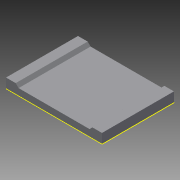
# Autodesk Inventor part: base
Saved by Autodesk Inventor 2016 (Build 200138000, 138)
## iProperties
Created: 2015-09-10
Part Number: base
Material: Gravel
Document SubType Name: Modeling
Designer: Students
Density: 1.84 g/cm^3
Appearance: Gravel - Compact
Author: Students
Autodesk Inventor part; units mm, degrees
ref_plane "YZ Plane" through (0, 0, 0) normal (1, 0, 0) x (0, 1, 0)
ref_plane "XZ Plane" through (0, 0, 0) normal (0, 1, 0) x (-1, 0, 0)
ref_plane "XY Plane" through (0, 0, 0) normal (0, 0, 1) x (1, 0, 0)
sketch "Sketch1" plane through (0, 0, 0) normal (0, 1, 0) x (-1, 0, 0)
  line L0 (100, 0) -> (100, -10)
  line L1 (100, -10) -> (0, -10)
  line L2 (0, -10) -> (0, 0)
  line L3 (0, 0) -> (10, 0)
  line L4 (13, -3) -> (10, 0)
  line L5 (86.9207, -3) -> (89.9207, 0)
  line L6 (13, -3) -> (86.9207, -3)
  line L7 (0, 0) -> (10, 0)
  line L8 (89.9207, 0) -> (100, 0)
  point P0 (13, 0)
  point P1 (13, 0)
  point P2 (89.9207, 0)
  point P3 (89.9207, 0)
  point P4 (86.9207, 0)
  constraints: 18 end point, 8 coincident, 5 parallel, 3 perpendicular, 2 horizontal
extrude "Extrusion1" add sketch "Sketch1" along normal blind 75
sketch "Sketch2" plane through (0, 0, -10) normal (0, 0, -1) x (-1, 0, 0)
  line L0 (0, 0) -> (100, 0) projected
  line L1 (100, 0) -> (100, 75) projected
  line L2 (0, 75) -> (100, 75) projected
  line L3 (0, 0) -> (0, 75) projected
body "Solid1"
